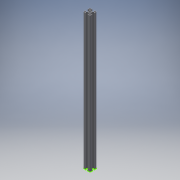
# Autodesk Inventor part: 3030 600mm
Saved by Autodesk Inventor 2017 (Build 210142000, 142)
## iProperties
Created: 2016-06-13
Part Number: 3030 600mm
Material: Generic
Document SubType Name: Modeling
Designer: joshmamo
Density: 1 g/cm^3
Appearance: Default
Author: joshmamo
Autodesk Inventor part; units mm, degrees
ref_plane "YZ Plane" through (0, 0, 0) normal (1, 0, 0) x (0, 1, 0)
ref_plane "XZ Plane" through (0, 0, 0) normal (0, 1, 0) x (-1, 0, 0)
ref_plane "XY Plane" through (0, 0, 0) normal (0, 0, 1) x (1, 0, 0)
sketch "Sketch1" plane through (0, 0, 0) normal (0, 0, 1) x (1, 0, 0)
  arc A0 (9.881, 13.6999) -> (9.5, 13.3189) centre (9.881, 13.3189) ccw
  line L0 (12.6999, 13.6999) -> (9.881, 13.6999)
  arc A1 (13.6999, 12.6999) -> (12.6999, 13.6999) centre (12.6999, 12.6999) ccw
  line L1 (13.6999, 9.881) -> (13.6999, 12.6999)
  arc A2 (13.3189, 9.5) -> (13.6999, 9.881) centre (13.3189, 9.881) ccw
  line L2 (9.88, 9.5) -> (13.3189, 9.5)
  arc A3 (9.5, 9.88) -> (9.88, 9.5) centre (9.88, 9.88) ccw
  line L3 (9.5, 13.3189) -> (9.5, 9.88)
  arc A4 (-9.5, 13.3189) -> (-9.881, 13.6999) centre (-9.881, 13.3189) ccw
  line L4 (-9.5, 9.88) -> (-9.5, 13.3189)
  arc A5 (-9.88, 9.5) -> (-9.5, 9.88) centre (-9.88, 9.88) ccw
  line L5 (-13.3189, 9.5) -> (-9.88, 9.5)
  arc A6 (-13.6999, 9.881) -> (-13.3189, 9.5) centre (-13.3189, 9.881) ccw
  line L6 (-13.6999, 12.6999) -> (-13.6999, 9.881)
  arc A7 (-12.6999, 13.6999) -> (-13.6999, 12.6999) centre (-12.6999, 12.6999) ccw
  line L7 (-9.881, 13.6999) -> (-12.6999, 13.6999)
  arc A8 (-1.4942, -3.1981) -> (1.4942, -3.1981) centre (0, 0) ccw
  line L8 (-2.4733, -3.9799) -> (-1.4942, -3.1981)
  arc A9 (-3.9799, -2.4733) -> (-2.4733, -3.9799) centre (-3.1422, -3.1422) ccw
  line L9 (-3.1981, -1.4942) -> (-3.9799, -2.4733)
  arc A10 (-3.1981, 1.4942) -> (-3.1981, -1.4942) centre (0, 0) ccw
  line L10 (-3.9799, 2.4733) -> (-3.1981, 1.4942)
  arc A11 (-2.4733, 3.9799) -> (-3.9799, 2.4733) centre (-3.1422, 3.1422) ccw
  line L11 (-1.4942, 3.1981) -> (-2.4733, 3.9799)
  arc A12 (1.4942, 3.1981) -> (-1.4942, 3.1981) centre (0, 0) ccw
  line L12 (2.4733, 3.9799) -> (1.4942, 3.1981)
  arc A13 (3.9799, 2.4733) -> (2.4733, 3.9799) centre (3.1422, 3.1422) ccw
  line L13 (3.1981, 1.4942) -> (3.9799, 2.4733)
  arc A14 (3.1981, -1.4942) -> (3.1981, 1.4942) centre (0, 0) ccw
  line L14 (3.9799, -2.4733) -> (3.1981, -1.4942)
  arc A15 (2.4733, -3.9799) -> (3.9799, -2.4733) centre (3.1422, -3.1422) ccw
  line L15 (1.4942, -3.1981) -> (2.4733, -3.9799)
  arc A16 (-13.3189, -9.5) -> (-13.6999, -9.881) centre (-13.3189, -9.881) ccw
  line L16 (-9.88, -9.5) -> (-13.3189, -9.5)
  arc A17 (-9.5, -9.88) -> (-9.88, -9.5) centre (-9.88, -9.88) ccw
  line L17 (-9.5, -13.3189) -> (-9.5, -9.88)
  arc A18 (-9.881, -13.6999) -> (-9.5, -13.3189) centre (-9.881, -13.3189) ccw
  line L18 (-12.6999, -13.6999) -> (-9.881, -13.6999)
  arc A19 (-13.6999, -12.6999) -> (-12.6999, -13.6999) centre (-12.6999, -12.6999) ccw
  line L19 (-13.6999, -9.881) -> (-13.6999, -12.6999)
  arc A20 (9.5, -13.3189) -> (9.881, -13.6999) centre (9.881, -13.3189) ccw
  line L20 (9.5, -9.88) -> (9.5, -13.3189)
  arc A21 (9.88, -9.5) -> (9.5, -9.88) centre (9.88, -9.88) ccw
  line L21 (13.3189, -9.5) -> (9.88, -9.5)
  arc A22 (13.6999, -9.881) -> (13.3189, -9.5) centre (13.3189, -9.881) ccw
  line L22 (13.6999, -12.6999) -> (13.6999, -9.881)
  arc A23 (12.6999, -13.6999) -> (13.6999, -12.6999) centre (12.6999, -12.6999) ccw
  line L23 (9.881, -13.6999) -> (12.6999, -13.6999)
  arc A24 (13.2425, -4) -> (12.7425, -4.5) centre (13.2425, -4.5) ccw
  line L24 (12.7425, -4.5) -> (12.7425, -7.7325)
  arc A25 (12.2428, -8.25) -> (12.7425, -7.7325) centre (12.2428, -7.75) ccw
  line L25 (12.2428, -8.25) -> (10.2602, -8.25)
  arc A26 (9.9066, -8.1035) -> (10.2602, -8.25) centre (10.2602, -7.75) ccw
  line L26 (9.9066, -8.1035) -> (5.9811, -4.178)
  arc A27 (5.8347, -3.8245) -> (5.9811, -4.178) centre (6.3347, -3.8245) ccw
  line L27 (5.8347, -3.8245) -> (5.8347, -1.0125)
  line L28 (5.8347, -1.0125) -> (5.3247, -0.0625)
  line L29 (5.3247, -0.0625) -> (5.8347, 0.8875)
  line L30 (5.8347, 0.8875) -> (5.8347, 3.8245)
  arc A28 (5.9811, 4.178) -> (5.8347, 3.8245) centre (6.3347, 3.8245) ccw
  line L31 (5.9811, 4.178) -> (9.9066, 8.1035)
  arc A29 (10.2602, 8.25) -> (9.9066, 8.1035) centre (10.2602, 7.75) ccw
  line L32 (10.2602, 8.25) -> (12.2428, 8.25)
  arc A30 (12.7425, 7.7325) -> (12.2428, 8.25) centre (12.2428, 7.75) ccw
  line L33 (12.7425, 7.7325) -> (12.7425, 4.5)
  arc A31 (12.7425, 4.5) -> (13.2425, 4) centre (13.2425, 4.5) ccw
  line L34 (13.2425, 4) -> (14.4999, 4)
  arc A32 (14.4999, 4) -> (14.9999, 4.5) centre (14.4999, 4.5) ccw
  line L35 (14.9999, 4.5) -> (14.9999, 12.9999)
  arc A33 (14.9999, 12.9999) -> (12.9999, 14.9999) centre (12.9999, 12.9999) ccw
  line L36 (12.9999, 14.9999) -> (4.5, 14.9999)
  arc A34 (4.5, 14.9999) -> (4, 14.4999) centre (4.5, 14.4999) ccw
  line L37 (4, 14.4999) -> (4, 13.2425)
  arc A35 (4, 13.2425) -> (4.5, 12.7425) centre (4.5, 13.2425) ccw
  line L38 (4.5, 12.7425) -> (7.7325, 12.7425)
  arc A36 (8.25, 12.2428) -> (7.7325, 12.7425) centre (7.75, 12.2428) ccw
  line L39 (8.25, 12.2428) -> (8.25, 10.2602)
  arc A37 (8.1035, 9.9066) -> (8.25, 10.2602) centre (7.75, 10.2602) ccw
  line L40 (8.1035, 9.9066) -> (4.178, 5.9811)
  arc A38 (3.8245, 5.8347) -> (4.178, 5.9811) centre (3.8245, 6.3347) ccw
  line L41 (3.8245, 5.8347) -> (0.95, 5.8347)
  line L42 (0.95, 5.8347) -> (0, 5.3247)
  line L43 (0, 5.3247) -> (-0.95, 5.8347)
  line L44 (-0.95, 5.8347) -> (-3.8245, 5.8347)
  arc A39 (-4.178, 5.9811) -> (-3.8245, 5.8347) centre (-3.8245, 6.3347) ccw
  line L45 (-4.178, 5.9811) -> (-8.1035, 9.9066)
  arc A40 (-8.25, 10.2602) -> (-8.1035, 9.9066) centre (-7.75, 10.2602) ccw
  line L46 (-8.25, 10.2602) -> (-8.25, 12.2428)
  arc A41 (-7.7325, 12.7425) -> (-8.25, 12.2428) centre (-7.75, 12.2428) ccw
  line L47 (-7.7325, 12.7425) -> (-4.5, 12.7425)
  arc A42 (-4.5, 12.7425) -> (-4, 13.2425) centre (-4.5, 13.2425) ccw
  line L48 (-4, 13.2425) -> (-4, 14.4999)
  arc A43 (-4, 14.4999) -> (-4.5, 14.9999) centre (-4.5, 14.4999) ccw
  line L49 (-4.5, 14.9999) -> (-12.9999, 14.9999)
  arc A44 (-12.9999, 14.9999) -> (-14.9999, 12.9999) centre (-12.9999, 12.9999) ccw
  line L50 (-14.9999, 12.9999) -> (-14.9999, 4.5)
  arc A45 (-14.9999, 4.5) -> (-14.4999, 4) centre (-14.4999, 4.5) ccw
  line L51 (-14.4999, 4) -> (-13.2425, 4)
  arc A46 (-13.2425, 4) -> (-12.7425, 4.5) centre (-13.2425, 4.5) ccw
  line L52 (-12.7425, 4.5) -> (-12.7425, 7.7325)
  arc A47 (-12.2428, 8.25) -> (-12.7425, 7.7325) centre (-12.2428, 7.75) ccw
  line L53 (-12.2428, 8.25) -> (-10.2602, 8.25)
  arc A48 (-9.9066, 8.1035) -> (-10.2602, 8.25) centre (-10.2602, 7.75) ccw
  line L54 (-9.9066, 8.1035) -> (-5.9811, 4.178)
  arc A49 (-5.8347, 3.8245) -> (-5.9811, 4.178) centre (-6.3347, 3.8245) ccw
  line L55 (-5.8347, 3.8245) -> (-5.8347, 0.8875)
  line L56 (-5.8347, 0.8875) -> (-5.3247, -0.0625)
  line L57 (-5.3247, -0.0625) -> (-5.8347, -1.0125)
  line L58 (-5.8347, -1.0125) -> (-5.8347, -3.8245)
  arc A50 (-5.9811, -4.178) -> (-5.8347, -3.8245) centre (-6.3347, -3.8245) ccw
  line L59 (-5.9811, -4.178) -> (-9.9066, -8.1035)
  arc A51 (-10.2602, -8.25) -> (-9.9066, -8.1035) centre (-10.2602, -7.75) ccw
  line L60 (-10.2602, -8.25) -> (-12.2428, -8.25)
  arc A52 (-12.7425, -7.7325) -> (-12.2428, -8.25) centre (-12.2428, -7.75) ccw
  line L61 (-12.7425, -7.7325) -> (-12.7425, -4.5)
  arc A53 (-12.7425, -4.5) -> (-13.2425, -4) centre (-13.2425, -4.5) ccw
  line L62 (-13.2425, -4) -> (-14.4999, -4)
  arc A54 (-14.4999, -4) -> (-14.9999, -4.5) centre (-14.4999, -4.5) ccw
  line L63 (-14.9999, -4.5) -> (-14.9999, -12.9999)
  arc A55 (-14.9999, -12.9999) -> (-12.9999, -14.9999) centre (-12.9999, -12.9999) ccw
  line L64 (-12.9999, -14.9999) -> (-4.5, -14.9999)
  arc A56 (-4.5, -14.9999) -> (-4, -14.4999) centre (-4.5, -14.4999) ccw
  line L65 (-4, -14.4999) -> (-4, -13.2425)
  arc A57 (-4, -13.2425) -> (-4.5, -12.7425) centre (-4.5, -13.2425) ccw
  line L66 (-4.5, -12.7425) -> (-7.7325, -12.7425)
  arc A58 (-8.25, -12.2428) -> (-7.7325, -12.7425) centre (-7.75, -12.2428) ccw
  line L67 (-8.25, -12.2428) -> (-8.25, -10.2602)
  arc A59 (-8.1035, -9.9066) -> (-8.25, -10.2602) centre (-7.75, -10.2602) ccw
  line L68 (-8.1035, -9.9066) -> (-4.178, -5.9811)
  arc A60 (-3.8245, -5.8347) -> (-4.178, -5.9811) centre (-3.8245, -6.3347) ccw
  line L69 (-3.8245, -5.8347) -> (-0.95, -5.8347)
  line L70 (-0.95, -5.8347) -> (0, -5.3247)
  line L71 (0, -5.3247) -> (0.95, -5.8347)
  line L72 (0.95, -5.8347) -> (3.8245, -5.8347)
  arc A61 (4.178, -5.9811) -> (3.8245, -5.8347) centre (3.8245, -6.3347) ccw
  line L73 (4.178, -5.9811) -> (8.1035, -9.9066)
  arc A62 (8.25, -10.2602) -> (8.1035, -9.9066) centre (7.75, -10.2602) ccw
  line L74 (8.25, -10.2602) -> (8.25, -12.2428)
  arc A63 (7.7325, -12.7425) -> (8.25, -12.2428) centre (7.75, -12.2428) ccw
  line L75 (7.7325, -12.7425) -> (4.5, -12.7425)
  arc A64 (4.5, -12.7425) -> (4, -13.2425) centre (4.5, -13.2425) ccw
  line L76 (4, -13.2425) -> (4, -14.4999)
  arc A65 (4, -14.4999) -> (4.5, -14.9999) centre (4.5, -14.4999) ccw
  line L77 (4.5, -14.9999) -> (12.9999, -14.9999)
  arc A66 (12.9999, -14.9999) -> (14.9999, -12.9999) centre (12.9999, -12.9999) ccw
  line L78 (14.9999, -12.9999) -> (14.9999, -4.5)
  arc A67 (14.9999, -4.5) -> (14.4999, -4) centre (14.4999, -4.5) ccw
  line L79 (14.4999, -4) -> (13.2425, -4)
  constraints: 160 end point, 136 point on circle, 68 centre point
sketch "Sketch3" plane through (0, 0, 0) normal (0, 0, 1) x (1, 0, 0)
  arc A0 (9.881, 13.6999) -> (9.5, 13.3189) centre (9.881, 13.3189) ccw
  line L0 (12.6999, 13.6999) -> (9.881, 13.6999)
  arc A1 (13.6999, 12.6999) -> (12.6999, 13.6999) centre (12.6999, 12.6999) ccw
  line L1 (13.6999, 9.881) -> (13.6999, 12.6999)
  arc A2 (13.3189, 9.5) -> (13.6999, 9.881) centre (13.3189, 9.881) ccw
  line L2 (9.88, 9.5) -> (13.3189, 9.5)
  arc A3 (9.5, 9.88) -> (9.88, 9.5) centre (9.88, 9.88) ccw
  line L3 (9.5, 13.3189) -> (9.5, 9.88)
  arc A4 (-9.5, 13.3189) -> (-9.881, 13.6999) centre (-9.881, 13.3189) ccw
  line L4 (-9.5, 9.88) -> (-9.5, 13.3189)
  arc A5 (-9.88, 9.5) -> (-9.5, 9.88) centre (-9.88, 9.88) ccw
  line L5 (-13.3189, 9.5) -> (-9.88, 9.5)
  arc A6 (-13.6999, 9.881) -> (-13.3189, 9.5) centre (-13.3189, 9.881) ccw
  line L6 (-13.6999, 12.6999) -> (-13.6999, 9.881)
  arc A7 (-12.6999, 13.6999) -> (-13.6999, 12.6999) centre (-12.6999, 12.6999) ccw
  line L7 (-9.881, 13.6999) -> (-12.6999, 13.6999)
  arc A8 (-1.4942, -3.1981) -> (1.4942, -3.1981) centre (0, 0) ccw
  line L8 (-2.4733, -3.9799) -> (-1.4942, -3.1981)
  arc A9 (-3.9799, -2.4733) -> (-2.4733, -3.9799) centre (-3.1422, -3.1422) ccw
  line L9 (-3.1981, -1.4942) -> (-3.9799, -2.4733)
  arc A10 (-3.1981, 1.4942) -> (-3.1981, -1.4942) centre (0, 0) ccw
  line L10 (-3.9799, 2.4733) -> (-3.1981, 1.4942)
  arc A11 (-2.4733, 3.9799) -> (-3.9799, 2.4733) centre (-3.1422, 3.1422) ccw
  line L11 (-1.4942, 3.1981) -> (-2.4733, 3.9799)
  arc A12 (1.4942, 3.1981) -> (-1.4942, 3.1981) centre (0, 0) ccw
  line L12 (2.4733, 3.9799) -> (1.4942, 3.1981)
  arc A13 (3.9799, 2.4733) -> (2.4733, 3.9799) centre (3.1422, 3.1422) ccw
  line L13 (3.1981, 1.4942) -> (3.9799, 2.4733)
  arc A14 (3.1981, -1.4942) -> (3.1981, 1.4942) centre (0, 0) ccw
  line L14 (3.9799, -2.4733) -> (3.1981, -1.4942)
  arc A15 (2.4733, -3.9799) -> (3.9799, -2.4733) centre (3.1422, -3.1422) ccw
  line L15 (1.4942, -3.1981) -> (2.4733, -3.9799)
  arc A16 (-13.3189, -9.5) -> (-13.6999, -9.881) centre (-13.3189, -9.881) ccw
  line L16 (-9.88, -9.5) -> (-13.3189, -9.5)
  arc A17 (-9.5, -9.88) -> (-9.88, -9.5) centre (-9.88, -9.88) ccw
  line L17 (-9.5, -13.3189) -> (-9.5, -9.88)
  arc A18 (-9.881, -13.6999) -> (-9.5, -13.3189) centre (-9.881, -13.3189) ccw
  line L18 (-12.6999, -13.6999) -> (-9.881, -13.6999)
  arc A19 (-13.6999, -12.6999) -> (-12.6999, -13.6999) centre (-12.6999, -12.6999) ccw
  line L19 (-13.6999, -9.881) -> (-13.6999, -12.6999)
  arc A20 (9.5, -13.3189) -> (9.881, -13.6999) centre (9.881, -13.3189) ccw
  line L20 (9.5, -9.88) -> (9.5, -13.3189)
  arc A21 (9.88, -9.5) -> (9.5, -9.88) centre (9.88, -9.88) ccw
  line L21 (13.3189, -9.5) -> (9.88, -9.5)
  arc A22 (13.6999, -9.881) -> (13.3189, -9.5) centre (13.3189, -9.881) ccw
  line L22 (13.6999, -12.6999) -> (13.6999, -9.881)
  arc A23 (12.6999, -13.6999) -> (13.6999, -12.6999) centre (12.6999, -12.6999) ccw
  line L23 (9.881, -13.6999) -> (12.6999, -13.6999)
  arc A24 (13.2425, -4) -> (12.7425, -4.5) centre (13.2425, -4.5) ccw
  line L24 (12.7425, -4.5) -> (12.7425, -7.7325)
  arc A25 (12.2428, -8.25) -> (12.7425, -7.7325) centre (12.2428, -7.75) ccw
  line L25 (12.2428, -8.25) -> (10.2602, -8.25)
  arc A26 (9.9066, -8.1035) -> (10.2602, -8.25) centre (10.2602, -7.75) ccw
  line L26 (9.9066, -8.1035) -> (5.9811, -4.178)
  arc A27 (5.8347, -3.8245) -> (5.9811, -4.178) centre (6.3347, -3.8245) ccw
  line L27 (5.8347, -3.8245) -> (5.8347, -1.0125)
  line L28 (5.8347, -1.0125) -> (5.3247, -0.0625)
  line L29 (5.3247, -0.0625) -> (5.8347, 0.8875)
  line L30 (5.8347, 0.8875) -> (5.8347, 3.8245)
  arc A28 (5.9811, 4.178) -> (5.8347, 3.8245) centre (6.3347, 3.8245) ccw
  line L31 (5.9811, 4.178) -> (9.9066, 8.1035)
  arc A29 (10.2602, 8.25) -> (9.9066, 8.1035) centre (10.2602, 7.75) ccw
  line L32 (10.2602, 8.25) -> (12.2428, 8.25)
  arc A30 (12.7425, 7.7325) -> (12.2428, 8.25) centre (12.2428, 7.75) ccw
  line L33 (12.7425, 7.7325) -> (12.7425, 4.5)
  arc A31 (12.7425, 4.5) -> (13.2425, 4) centre (13.2425, 4.5) ccw
  line L34 (13.2425, 4) -> (14.4999, 4)
  arc A32 (14.4999, 4) -> (14.9999, 4.5) centre (14.4999, 4.5) ccw
  line L35 (14.9999, 4.5) -> (14.9999, 12.9999)
  arc A33 (14.9999, 12.9999) -> (12.9999, 14.9999) centre (12.9999, 12.9999) ccw
  line L36 (12.9999, 14.9999) -> (4.5, 14.9999)
  arc A34 (4.5, 14.9999) -> (4, 14.4999) centre (4.5, 14.4999) ccw
  line L37 (4, 14.4999) -> (4, 13.2425)
  arc A35 (4, 13.2425) -> (4.5, 12.7425) centre (4.5, 13.2425) ccw
  line L38 (4.5, 12.7425) -> (7.7325, 12.7425)
  arc A36 (8.25, 12.2428) -> (7.7325, 12.7425) centre (7.75, 12.2428) ccw
  line L39 (8.25, 12.2428) -> (8.25, 10.2602)
  arc A37 (8.1035, 9.9066) -> (8.25, 10.2602) centre (7.75, 10.2602) ccw
  line L40 (8.1035, 9.9066) -> (4.178, 5.9811)
  arc A38 (3.8245, 5.8347) -> (4.178, 5.9811) centre (3.8245, 6.3347) ccw
  line L41 (3.8245, 5.8347) -> (0.95, 5.8347)
  line L42 (0.95, 5.8347) -> (0, 5.3247)
  line L43 (0, 5.3247) -> (-0.95, 5.8347)
  line L44 (-0.95, 5.8347) -> (-3.8245, 5.8347)
  arc A39 (-4.178, 5.9811) -> (-3.8245, 5.8347) centre (-3.8245, 6.3347) ccw
  line L45 (-4.178, 5.9811) -> (-8.1035, 9.9066)
  arc A40 (-8.25, 10.2602) -> (-8.1035, 9.9066) centre (-7.75, 10.2602) ccw
  line L46 (-8.25, 10.2602) -> (-8.25, 12.2428)
  arc A41 (-7.7325, 12.7425) -> (-8.25, 12.2428) centre (-7.75, 12.2428) ccw
  line L47 (-7.7325, 12.7425) -> (-4.5, 12.7425)
  arc A42 (-4.5, 12.7425) -> (-4, 13.2425) centre (-4.5, 13.2425) ccw
  line L48 (-4, 13.2425) -> (-4, 14.4999)
  arc A43 (-4, 14.4999) -> (-4.5, 14.9999) centre (-4.5, 14.4999) ccw
  line L49 (-4.5, 14.9999) -> (-12.9999, 14.9999)
  arc A44 (-12.9999, 14.9999) -> (-14.9999, 12.9999) centre (-12.9999, 12.9999) ccw
  line L50 (-14.9999, 12.9999) -> (-14.9999, 4.5)
  arc A45 (-14.9999, 4.5) -> (-14.4999, 4) centre (-14.4999, 4.5) ccw
  line L51 (-14.4999, 4) -> (-13.2425, 4)
  arc A46 (-13.2425, 4) -> (-12.7425, 4.5) centre (-13.2425, 4.5) ccw
  line L52 (-12.7425, 4.5) -> (-12.7425, 7.7325)
  arc A47 (-12.2428, 8.25) -> (-12.7425, 7.7325) centre (-12.2428, 7.75) ccw
  line L53 (-12.2428, 8.25) -> (-10.2602, 8.25)
  arc A48 (-9.9066, 8.1035) -> (-10.2602, 8.25) centre (-10.2602, 7.75) ccw
  line L54 (-9.9066, 8.1035) -> (-5.9811, 4.178)
  arc A49 (-5.8347, 3.8245) -> (-5.9811, 4.178) centre (-6.3347, 3.8245) ccw
  line L55 (-5.8347, 3.8245) -> (-5.8347, 0.8875)
  line L56 (-5.8347, 0.8875) -> (-5.3247, -0.0625)
  line L57 (-5.3247, -0.0625) -> (-5.8347, -1.0125)
  line L58 (-5.8347, -1.0125) -> (-5.8347, -3.8245)
  arc A50 (-5.9811, -4.178) -> (-5.8347, -3.8245) centre (-6.3347, -3.8245) ccw
  line L59 (-5.9811, -4.178) -> (-9.9066, -8.1035)
  arc A51 (-10.2602, -8.25) -> (-9.9066, -8.1035) centre (-10.2602, -7.75) ccw
  line L60 (-10.2602, -8.25) -> (-12.2428, -8.25)
  arc A52 (-12.7425, -7.7325) -> (-12.2428, -8.25) centre (-12.2428, -7.75) ccw
  line L61 (-12.7425, -7.7325) -> (-12.7425, -4.5)
  arc A53 (-12.7425, -4.5) -> (-13.2425, -4) centre (-13.2425, -4.5) ccw
  line L62 (-13.2425, -4) -> (-14.4999, -4)
  arc A54 (-14.4999, -4) -> (-14.9999, -4.5) centre (-14.4999, -4.5) ccw
  line L63 (-14.9999, -4.5) -> (-14.9999, -12.9999)
  arc A55 (-14.9999, -12.9999) -> (-12.9999, -14.9999) centre (-12.9999, -12.9999) ccw
  line L64 (-12.9999, -14.9999) -> (-4.5, -14.9999)
  arc A56 (-4.5, -14.9999) -> (-4, -14.4999) centre (-4.5, -14.4999) ccw
  line L65 (-4, -14.4999) -> (-4, -13.2425)
  arc A57 (-4, -13.2425) -> (-4.5, -12.7425) centre (-4.5, -13.2425) ccw
  line L66 (-4.5, -12.7425) -> (-7.7325, -12.7425)
  arc A58 (-8.25, -12.2428) -> (-7.7325, -12.7425) centre (-7.75, -12.2428) ccw
  line L67 (-8.25, -12.2428) -> (-8.25, -10.2602)
  arc A59 (-8.1035, -9.9066) -> (-8.25, -10.2602) centre (-7.75, -10.2602) ccw
  line L68 (-8.1035, -9.9066) -> (-4.178, -5.9811)
  arc A60 (-3.8245, -5.8347) -> (-4.178, -5.9811) centre (-3.8245, -6.3347) ccw
  line L69 (-3.8245, -5.8347) -> (-0.95, -5.8347)
  line L70 (-0.95, -5.8347) -> (0, -5.3247)
  line L71 (0, -5.3247) -> (0.95, -5.8347)
  line L72 (0.95, -5.8347) -> (3.8245, -5.8347)
  arc A61 (4.178, -5.9811) -> (3.8245, -5.8347) centre (3.8245, -6.3347) ccw
  line L73 (4.178, -5.9811) -> (8.1035, -9.9066)
  arc A62 (8.25, -10.2602) -> (8.1035, -9.9066) centre (7.75, -10.2602) ccw
  line L74 (8.25, -10.2602) -> (8.25, -12.2428)
  arc A63 (7.7325, -12.7425) -> (8.25, -12.2428) centre (7.75, -12.2428) ccw
  line L75 (7.7325, -12.7425) -> (4.5, -12.7425)
  arc A64 (4.5, -12.7425) -> (4, -13.2425) centre (4.5, -13.2425) ccw
  line L76 (4, -13.2425) -> (4, -14.4999)
  arc A65 (4, -14.4999) -> (4.5, -14.9999) centre (4.5, -14.4999) ccw
  line L77 (4.5, -14.9999) -> (12.9999, -14.9999)
  arc A66 (12.9999, -14.9999) -> (14.9999, -12.9999) centre (12.9999, -12.9999) ccw
  line L78 (14.9999, -12.9999) -> (14.9999, -4.5)
  arc A67 (14.9999, -4.5) -> (14.4999, -4) centre (14.4999, -4.5) ccw
  line L79 (14.4999, -4) -> (13.2425, -4)
  constraints: 160 end point, 136 point on circle, 68 centre point, 1 coincident
extrude "Extrusion1" add sketch "Sketch3" along normal blind 600
ref_plane "Work Plane1" through (-17.9999, -135.9777, 660) normal (0, 0, 1) x (1, 0, 0)
body "Solid1"
